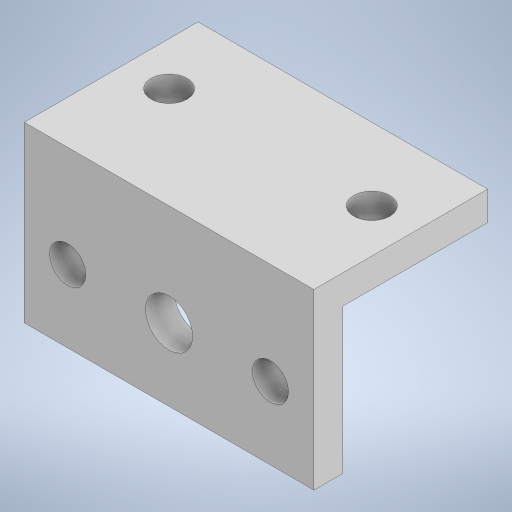
# Autodesk Inventor part: linac_lower_ax_mount_2
Saved by Autodesk Inventor 2024 (Build 280153000, 153)
## iProperties
Created: 2025-12-26
Part Number: linac_lower_ax_mount_2
Material: Generic
Document SubType Name: Modeling
Designer: schar
Density: 1 g/cm^3
Appearance: Default
Author: schar
Autodesk Inventor part; units mm, degrees
ref_plane "YZ Plane" through (0, 0, 0) normal (1, 0, 0) x (0, 1, 0)
ref_plane "XZ Plane" through (0, 0, 0) normal (0, 1, 0) x (-1, 0, 0)
ref_plane "XY Plane" through (0, 0, 0) normal (0, 0, 1) x (1, 0, 0)
sketch "Sketch1" plane through (0, 0, 0) normal (1, 0, 0) x (0, 1, 0)
  line L0 (0, 0) -> (-20, 0)
  line L1 (-20, 0) -> (-20, -20)
  line L2 (-20, -20) -> (0, -20)
  line L3 (0, -20) -> (0, 0)
  line L4 (0, -20) -> (4, -20)
  line L5 (4, -20) -> (4, 0)
  line L6 (4, 0) -> (0, 0)
  line L7 (0, 0) -> (0, -20)
  line L8 (4, 0) -> (0, 0)
  line L9 (0, 0) -> (0, 4)
  line L10 (0, 4) -> (4, 4)
  line L11 (4, 4) -> (4, 0)
  line L12 (0, 4) -> (-20, 4)
  line L13 (-20, 4) -> (-20, 0)
  line L14 (-20, 0) -> (0, 0)
  line L15 (0, 0) -> (0, 4)
  dimension "d0" = 20
  dimension "d1" = 20
  dimension "d2" = 4
  dimension "d3" = 4
  constraints: 32 end point, 8 parallel, 4 horizontal, 4 perpendicular, 2 point on line
  measures "d0" distance of L2.end L1.end
  measures "d1" distance of L1.end L0.end
  measures "d2" distance of L6.end L5.end
  measures "d3" distance of L8.end L9.end
extrude "Extrusion1" add sketch "Sketch1" along normal blind 40 contours L6 L5 L4 L3 | L9 L10 L11 L6 | L0 L13 L12 L9
sketch "Sketch2" plane through (0, -20, 4) normal (0, 0, 1) x (1, 0, 0)
  line L0 (0, 0) -> (40, 0) projected
  line L1 (20, 0) -> (20, 10)
  circle A0 centre (20, 10) radius 3.25
  point P0 (0, 20)
  dimension "d6" = 10
  dimension "d7" = 6.5
  constraints: 2 end point, 1 centre point, 1 coincident, 1 midpoint, 1 vertical
  measures "d6" distance of L1.start L1.end
  measures "d7" diameter of A0
extrude "Extrusion2" cut sketch "Sketch2" against normal through all
sketch "Sketch3" plane through (0, -20, 4) normal (0, 0, 1) x (1, 0, 0)
  line L0 (0, 0) -> (40, 0) projected
  line L1 (0, 0) -> (6, 0)
  line L2 (6, 0) -> (6, 10)
  line L3 (0, 20) -> (40, 20) projected
  line L4 (20, 0) -> (20, 3.9788)
  line L5 (40, 0) -> (0, 0)
  line L6 (34, 0) -> (34, 10)
  circle A0 centre (34, 10) radius 2.5
  circle A1 centre (6, 10) radius 2.5
  dimension "d10" = 6
  dimension "d11" = 10
  dimension "d12" = 5
  dimension "d13" = 5
  constraints: 10 end point, 4 symmetric about line, 2 centre point, 2 coincident, 2 point on line, 1 midpoint, 1 perpendicular, 1 vertical
  measures "d10" distance of L0.start L1.end
  measures "d11" distance of L1.end L2.end
  measures "d12" diameter of A0
  measures "d13" diameter of A1
extrude "Extrusion3" cut sketch "Sketch3" against normal blind 10
sketch "Sketch4" plane through (0, 4, 4) normal (0, 1, 0) x (1, 0, 0)
  line L0 (0, 24) -> (40, 24) projected
  line L1 (0, 24) -> (6, 24)
  line L2 (6, 24) -> (6, 14)
  line L3 (40, 24) -> (34, 24)
  line L4 (34, 24) -> (34, 14)
  circle A0 centre (34, 14) radius 2.5
  circle A1 centre (6, 14) radius 2.5
  point P0 (0, 4)
  dimension "d16" = 6
  dimension "d17" = 10
  dimension "d18" = 6
  dimension "d19" = 10
  dimension "d20" = 5
  dimension "d21" = 5
  constraints: 8 end point, 2 centre point, 2 coincident, 2 perpendicular, 2 point on line
  measures "d16" distance of L0.start L1.end
  measures "d17" distance of L1.end L2.end
  measures "d18" distance of L0.end L3.end
  measures "d19" distance of L3.end L4.end
  measures "d20" diameter of A0
  measures "d21" diameter of A1
extrude "Extrusion4" cut sketch "Sketch4" against normal blind 10
body "Solid1"
